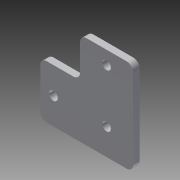
# Autodesk Inventor part: Spacer 2
Saved by Autodesk Inventor 2014 (Build 180170000, 170)
## iProperties
Created: 2014-01-17
Part Number: Spacer 2
Material: ABS Plastic
Document SubType Name: Modeling
Designer: Michael
Density: 1.06 g/cm^3
Appearance: Smooth - White
Author: Michael
Autodesk Inventor part; units mm, degrees
ref_plane "YZ Plane" through (0, 0, 0) normal (1, 0, 0) x (0, 1, 0)
ref_plane "XZ Plane" through (0, 0, 0) normal (0, 1, 0) x (-1, 0, 0)
ref_plane "XY Plane" through (0, 0, 0) normal (0, 0, 1) x (1, 0, 0)
sketch "Sketch1" plane through (0, 0, 0) normal (0, 0, 1) x (1, 0, 0)
  line L0 (0, 0) -> (44.45, 0)
  line L1 (44.45, 0) -> (44.45, 44.45)
  line L2 (44.45, 44.45) -> (19.05, 44.45)
  line L3 (19.05, 44.45) -> (19.05, 25.4)
  line L4 (19.05, 25.4) -> (0, 25.4)
  line L5 (0, 25.4) -> (0, 0)
  circle A0 centre (6.35, 12.7) radius 2.0701
  circle A1 centre (31.75, 12.7) radius 2.0701
  circle A2 centre (31.75, 38.1) radius 2.0701
  dimension "d0" = 44.45
  dimension "d1" = 25.4
  dimension "d2" = 4.1402
  dimension "d3" = 12.7
  dimension "d4" = 6.35
  dimension "d7" = 25.4
  dimension "d14" = 25.4
  constraints: 12 end point, 4 parallel, 3 centre point, 3 perpendicular, 2 horizontal, 1 vertical, 4 other
  measures "d0" distance of L0.start L0.end
  measures "d1" distance of L1.end L2.end
  measures "d2" diameter of A0
  measures "d3" distance from line of L0 A0.centre
  measures "d4" distance from line of L5 A0.centre
  measures "d7" distance of A0.centre A1.centre
  measures "d14" distance of A1.centre A2.centre
extrude "Extrusion1" add sketch "Sketch1" along normal blind 3.175
fillet "Fillet1" radius 3.175 6 edges at (19.05, 25.4, 1.5875) (0, 25.4, 1.5875) (0, 0, 1.5875) (44.45, 0, 1.5875) (44.45, 44.45, 1.5875) (19.05, 44.45, 1.5875)
body "Solid1"
